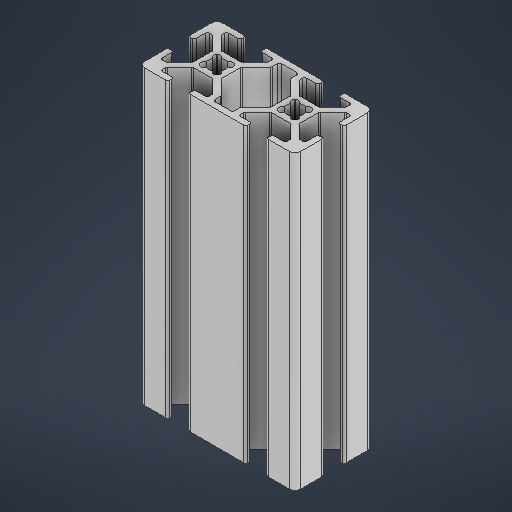
# Autodesk Inventor part: 20x40x100mm-Extrusion
Saved by Autodesk Inventor 2026.2 (Build 302298000, 298)
## iProperties
Created: 2026-06-17
Part Number: 20x40x100mm-Extrusion
Material: Aluminum 6061
Document SubType Name: Modeling
Designer: Kenji
Density: 2.7 g/cm^3
Appearance: Aluminum - Dark
Mass: 74.3604 g
Surface Area: 338.77 cm^2
Volume: 27.5409 cm^3
Author: Kenji
Autodesk Inventor part; units mm, degrees
ref_plane "YZ Plane" through (0, 0, 0) normal (1, 0, 0) x (0, 1, 0)
ref_plane "XZ Plane" through (0, 0, 0) normal (0, 1, 0) x (-1, 0, 0)
ref_plane "XY Plane" through (0, 0, 0) normal (0, 0, 1) x (1, 0, 0)
sketch "Sketch1" plane through (0, 0, 0) normal (0, 1, 0) x (-1, 0, 0)
  arc A0 (12.6651, -3.7453) -> (12.3059, -3.5965) centre (12.3059, -4.1045) ccw
  line L0 (15.7682, -6.8484) -> (12.6651, -3.7453)
  arc A1 (15.917, -7.2076) -> (15.7682, -6.8484) centre (15.409, -7.2076) ccw
  line L1 (15.917, -7.9335) -> (15.917, -7.2076)
  arc A2 (15.409, -8.4415) -> (15.917, -7.9335) centre (15.409, -7.9335) ccw
  line L2 (13.06, -8.4415) -> (15.409, -8.4415)
  arc A3 (13.06, -8.4415) -> (12.552, -8.9495) centre (13.06, -8.9495) ccw
  line L3 (12.552, -9.4335) -> (12.552, -8.9495)
  arc A4 (12.552, -9.4335) -> (13.06, -9.9415) centre (13.06, -9.4335) ccw
  line L4 (18.422, -9.9415) -> (13.06, -9.9415)
  arc A5 (18.422, -9.9415) -> (19.922, -8.4415) centre (18.422, -8.4415) ccw
  line L5 (19.922, -3.0795) -> (19.922, -8.4415)
  arc A6 (19.922, -3.0795) -> (19.414, -2.5715) centre (19.414, -3.0795) ccw
  line L6 (18.93, -2.5715) -> (19.414, -2.5715)
  arc A7 (18.93, -2.5715) -> (18.422, -3.0795) centre (18.93, -3.0795) ccw
  line L7 (18.422, -5.4285) -> (18.422, -3.0795)
  arc A8 (17.914, -5.9365) -> (18.422, -5.4285) centre (17.914, -5.4285) ccw
  line L8 (17.1881, -5.9365) -> (17.914, -5.9365)
  arc A9 (16.8289, -5.7877) -> (17.1881, -5.9365) centre (17.1881, -5.4285) ccw
  line L9 (13.7258, -2.6846) -> (16.8289, -5.7877)
  arc A10 (13.577, -2.3254) -> (13.7258, -2.6846) centre (14.085, -2.3254) ccw
  line L10 (13.577, 2.4424) -> (13.577, -2.3254)
  arc A11 (13.7258, 2.8016) -> (13.577, 2.4424) centre (14.085, 2.4424) ccw
  line L11 (16.8289, 5.9047) -> (13.7258, 2.8016)
  arc A12 (17.1881, 6.0535) -> (16.8289, 5.9047) centre (17.1881, 5.5455) ccw
  line L12 (17.914, 6.0535) -> (17.1881, 6.0535)
  arc A13 (18.422, 5.5455) -> (17.914, 6.0535) centre (17.914, 5.5455) ccw
  line L13 (18.422, 3.1965) -> (18.422, 5.5455)
  arc A14 (18.422, 3.1965) -> (18.93, 2.6885) centre (18.93, 3.1965) ccw
  line L14 (19.414, 2.6885) -> (18.93, 2.6885)
  arc A15 (19.414, 2.6885) -> (19.922, 3.1965) centre (19.414, 3.1965) ccw
  line L15 (19.922, 8.5585) -> (19.922, 3.1965)
  arc A16 (19.922, 8.5585) -> (18.422, 10.0585) centre (18.422, 8.5585) ccw
  line L16 (13.06, 10.0585) -> (18.422, 10.0585)
  arc A17 (13.06, 10.0585) -> (12.552, 9.5505) centre (13.06, 9.5505) ccw
  line L17 (12.552, 9.0665) -> (12.552, 9.5505)
  arc A18 (12.552, 9.0665) -> (13.06, 8.5585) centre (13.06, 9.0665) ccw
  line L18 (15.409, 8.5585) -> (13.06, 8.5585)
  arc A19 (15.917, 8.0505) -> (15.409, 8.5585) centre (15.409, 8.0505) ccw
  line L19 (15.917, 7.3246) -> (15.917, 8.0505)
  arc A20 (15.7682, 6.9654) -> (15.917, 7.3246) centre (15.409, 7.3246) ccw
  line L20 (12.6651, 3.8623) -> (15.7682, 6.9654)
  arc A21 (12.3059, 3.7135) -> (12.6651, 3.8623) centre (12.3059, 4.2215) ccw
  line L21 (7.5381, 3.7135) -> (12.3059, 3.7135)
  arc A22 (7.1789, 3.8623) -> (7.5381, 3.7135) centre (7.5381, 4.2215) ccw
  line L22 (4.0758, 6.9654) -> (7.1789, 3.8623)
  arc A23 (3.927, 7.3246) -> (4.0758, 6.9654) centre (4.435, 7.3246) ccw
  line L23 (3.927, 8.0505) -> (3.927, 7.3246)
  arc A24 (4.435, 8.5585) -> (3.927, 8.0505) centre (4.435, 8.0505) ccw
  line L24 (6.784, 8.5585) -> (4.435, 8.5585)
  arc A25 (6.784, 8.5585) -> (7.292, 9.0665) centre (6.784, 9.0665) ccw
  line L25 (7.292, 9.5505) -> (7.292, 9.0665)
  arc A26 (7.292, 9.5505) -> (6.784, 10.0585) centre (6.784, 9.5505) ccw
  line L26 (-6.94, 10.0585) -> (6.784, 10.0585)
  arc A27 (-6.94, 10.0585) -> (-7.448, 9.5505) centre (-6.94, 9.5505) ccw
  line L27 (-7.448, 9.0665) -> (-7.448, 9.5505)
  arc A28 (-7.448, 9.0665) -> (-6.94, 8.5585) centre (-6.94, 9.0665) ccw
  line L28 (-4.591, 8.5585) -> (-6.94, 8.5585)
  arc A29 (-4.083, 8.0505) -> (-4.591, 8.5585) centre (-4.591, 8.0505) ccw
  line L29 (-4.083, 7.3246) -> (-4.083, 8.0505)
  arc A30 (-4.2318, 6.9654) -> (-4.083, 7.3246) centre (-4.591, 7.3246) ccw
  line L30 (-7.3349, 3.8623) -> (-4.2318, 6.9654)
  arc A31 (-7.6941, 3.7135) -> (-7.3349, 3.8623) centre (-7.6941, 4.2215) ccw
  line L31 (-12.4619, 3.7135) -> (-7.6941, 3.7135)
  arc A32 (-12.8211, 3.8623) -> (-12.4619, 3.7135) centre (-12.4619, 4.2215) ccw
  line L32 (-15.9242, 6.9654) -> (-12.8211, 3.8623)
  arc A33 (-16.073, 7.3246) -> (-15.9242, 6.9654) centre (-15.565, 7.3246) ccw
  line L33 (-16.073, 8.0505) -> (-16.073, 7.3246)
  arc A34 (-15.565, 8.5585) -> (-16.073, 8.0505) centre (-15.565, 8.0505) ccw
  line L34 (-13.216, 8.5585) -> (-15.565, 8.5585)
  arc A35 (-13.216, 8.5585) -> (-12.708, 9.0665) centre (-13.216, 9.0665) ccw
  line L35 (-12.708, 9.5505) -> (-12.708, 9.0665)
  arc A36 (-12.708, 9.5505) -> (-13.216, 10.0585) centre (-13.216, 9.5505) ccw
  line L36 (-18.578, 10.0585) -> (-13.216, 10.0585)
  arc A37 (-18.578, 10.0585) -> (-20.078, 8.5585) centre (-18.578, 8.5585) ccw
  line L37 (-20.078, 3.1965) -> (-20.078, 8.5585)
  arc A38 (-20.078, 3.1965) -> (-19.57, 2.6885) centre (-19.57, 3.1965) ccw
  line L38 (-19.086, 2.6885) -> (-19.57, 2.6885)
  arc A39 (-19.086, 2.6885) -> (-18.578, 3.1965) centre (-19.086, 3.1965) ccw
  line L39 (-18.578, 5.5455) -> (-18.578, 3.1965)
  arc A40 (-18.07, 6.0535) -> (-18.578, 5.5455) centre (-18.07, 5.5455) ccw
  line L40 (-17.3441, 6.0535) -> (-18.07, 6.0535)
  arc A41 (-16.9849, 5.9047) -> (-17.3441, 6.0535) centre (-17.3441, 5.5455) ccw
  line L41 (-13.8818, 2.8016) -> (-16.9849, 5.9047)
  arc A42 (-13.733, 2.4424) -> (-13.8818, 2.8016) centre (-14.241, 2.4424) ccw
  line L42 (-13.733, -2.3254) -> (-13.733, 2.4424)
  arc A43 (-13.8818, -2.6846) -> (-13.733, -2.3254) centre (-14.241, -2.3254) ccw
  line L43 (-16.9849, -5.7877) -> (-13.8818, -2.6846)
  arc A44 (-17.3441, -5.9365) -> (-16.9849, -5.7877) centre (-17.3441, -5.4285) ccw
  line L44 (-18.07, -5.9365) -> (-17.3441, -5.9365)
  arc A45 (-18.578, -5.4285) -> (-18.07, -5.9365) centre (-18.07, -5.4285) ccw
  line L45 (-18.578, -3.0795) -> (-18.578, -5.4285)
  arc A46 (-18.578, -3.0795) -> (-19.086, -2.5715) centre (-19.086, -3.0795) ccw
  line L46 (-19.57, -2.5715) -> (-19.086, -2.5715)
  arc A47 (-19.57, -2.5715) -> (-20.078, -3.0795) centre (-19.57, -3.0795) ccw
  line L47 (-20.078, -8.4415) -> (-20.078, -3.0795)
  arc A48 (-20.078, -8.4415) -> (-18.578, -9.9415) centre (-18.578, -8.4415) ccw
  line L48 (-13.216, -9.9415) -> (-18.578, -9.9415)
  arc A49 (-13.216, -9.9415) -> (-12.708, -9.4335) centre (-13.216, -9.4335) ccw
  line L49 (-12.708, -8.9495) -> (-12.708, -9.4335)
  arc A50 (-12.708, -8.9495) -> (-13.216, -8.4415) centre (-13.216, -8.9495) ccw
  line L50 (-15.565, -8.4415) -> (-13.216, -8.4415)
  arc A51 (-16.073, -7.9335) -> (-15.565, -8.4415) centre (-15.565, -7.9335) ccw
  line L51 (-16.073, -7.2076) -> (-16.073, -7.9335)
  arc A52 (-15.9242, -6.8484) -> (-16.073, -7.2076) centre (-15.565, -7.2076) ccw
  line L52 (-12.8211, -3.7453) -> (-15.9242, -6.8484)
  arc A53 (-12.4619, -3.5965) -> (-12.8211, -3.7453) centre (-12.4619, -4.1045) ccw
  line L53 (-7.6941, -3.5965) -> (-12.4619, -3.5965)
  arc A54 (-7.3349, -3.7453) -> (-7.6941, -3.5965) centre (-7.6941, -4.1045) ccw
  line L54 (-4.2318, -6.8484) -> (-7.3349, -3.7453)
  arc A55 (-4.083, -7.2076) -> (-4.2318, -6.8484) centre (-4.591, -7.2076) ccw
  line L55 (-4.083, -7.9335) -> (-4.083, -7.2076)
  arc A56 (-4.591, -8.4415) -> (-4.083, -7.9335) centre (-4.591, -7.9335) ccw
  line L56 (-6.94, -8.4415) -> (-4.591, -8.4415)
  arc A57 (-6.94, -8.4415) -> (-7.448, -8.9495) centre (-6.94, -8.9495) ccw
  line L57 (-7.448, -9.4335) -> (-7.448, -8.9495)
  arc A58 (-7.448, -9.4335) -> (-6.94, -9.9415) centre (-6.94, -9.4335) ccw
  line L58 (6.784, -9.9415) -> (-6.94, -9.9415)
  arc A59 (6.784, -9.9415) -> (7.292, -9.4335) centre (6.784, -9.4335) ccw
  line L59 (7.292, -8.9495) -> (7.292, -9.4335)
  arc A60 (7.292, -8.9495) -> (6.784, -8.4415) centre (6.784, -8.9495) ccw
  line L60 (4.435, -8.4415) -> (6.784, -8.4415)
  arc A61 (3.927, -7.9335) -> (4.435, -8.4415) centre (4.435, -7.9335) ccw
  line L61 (3.927, -7.2076) -> (3.927, -7.9335)
  arc A62 (4.0758, -6.8484) -> (3.927, -7.2076) centre (4.435, -7.2076) ccw
  line L62 (7.1789, -3.7453) -> (4.0758, -6.8484)
  arc A63 (7.5381, -3.5965) -> (7.1789, -3.7453) centre (7.5381, -4.1045) ccw
  line L63 (12.3059, -3.5965) -> (7.5381, -3.5965)
  arc A64 (-9.274, -1.8766) -> (-7.9531, -2.246) centre (-8.5096, -1.6895) ccw
  arc A65 (-10.882, -1.8766) -> (-9.274, -1.8766) centre (-10.078, 0.0585) ccw
  arc A66 (-12.2029, -2.246) -> (-10.882, -1.8766) centre (-11.6464, -1.6895) ccw
  line L64 (-12.2029, -2.246) -> (-12.3825, -2.0664)
  arc A67 (-12.0131, -0.7455) -> (-12.3825, -2.0664) centre (-11.826, -1.5099) ccw
  arc A68 (-12.0131, 0.8625) -> (-12.0131, -0.7455) centre (-10.078, 0.0585) ccw
  arc A69 (-12.3825, 2.1834) -> (-12.0131, 0.8625) centre (-11.826, 1.6269) ccw
  line L65 (-12.3825, 2.1834) -> (-12.2029, 2.363)
  arc A70 (-10.882, 1.9936) -> (-12.2029, 2.363) centre (-11.6464, 1.8065) ccw
  arc A71 (-9.274, 1.9936) -> (-10.882, 1.9936) centre (-10.078, 0.0585) ccw
  arc A72 (-7.9531, 2.363) -> (-9.274, 1.9936) centre (-8.5096, 1.8065) ccw
  line L66 (-7.9531, 2.363) -> (-7.7735, 2.1834)
  arc A73 (-8.1429, 0.8625) -> (-7.7735, 2.1834) centre (-8.33, 1.6269) ccw
  arc A74 (-8.1429, -0.7455) -> (-8.1429, 0.8625) centre (-10.078, 0.0585) ccw
  arc A75 (-7.7735, -2.0664) -> (-8.1429, -0.7455) centre (-8.33, -1.5099) ccw
  line L67 (-7.7735, -2.0664) -> (-7.9531, -2.246)
  arc A76 (10.726, -1.8766) -> (12.0469, -2.246) centre (11.4904, -1.6895) ccw
  arc A77 (9.118, -1.8766) -> (10.726, -1.8766) centre (9.922, 0.0585) ccw
  arc A78 (7.7971, -2.246) -> (9.118, -1.8766) centre (8.3536, -1.6895) ccw
  line L68 (7.7971, -2.246) -> (7.6175, -2.0664)
  arc A79 (7.9869, -0.7455) -> (7.6175, -2.0664) centre (8.174, -1.5099) ccw
  arc A80 (7.9869, 0.8625) -> (7.9869, -0.7455) centre (9.922, 0.0585) ccw
  arc A81 (7.6175, 2.1834) -> (7.9869, 0.8625) centre (8.174, 1.6269) ccw
  line L69 (7.6175, 2.1834) -> (7.7971, 2.363)
  arc A82 (9.118, 1.9936) -> (7.7971, 2.363) centre (8.3536, 1.8065) ccw
  arc A83 (10.726, 1.9936) -> (9.118, 1.9936) centre (9.922, 0.0585) ccw
  arc A84 (12.0469, 2.363) -> (10.726, 1.9936) centre (11.4904, 1.8065) ccw
  line L70 (12.0469, 2.363) -> (12.2265, 2.1834)
  arc A85 (11.8571, 0.8625) -> (12.2265, 2.1834) centre (11.67, 1.6269) ccw
  arc A86 (11.8571, -0.7455) -> (11.8571, 0.8625) centre (9.922, 0.0585) ccw
  arc A87 (12.2265, -2.0664) -> (11.8571, -0.7455) centre (11.67, -1.5099) ccw
  line L71 (12.2265, -2.0664) -> (12.0469, -2.246)
  arc A88 (1.919, -8.4415) -> (2.427, -7.9335) centre (1.919, -7.9335) ccw
  line L72 (1.919, -8.4415) -> (-2.075, -8.4415)
  arc A89 (-2.583, -7.9335) -> (-2.075, -8.4415) centre (-2.075, -7.9335) ccw
  line L73 (-2.583, -7.9335) -> (-2.583, -6.5863)
  arc A90 (-2.583, -6.5863) -> (-2.7318, -6.227) centre (-3.091, -6.5863) ccw
  line L74 (-2.7318, -6.227) -> (-6.2742, -2.6846)
  arc A91 (-6.423, -2.3254) -> (-6.2742, -2.6846) centre (-5.915, -2.3254) ccw
  line L75 (-6.423, -2.3254) -> (-6.423, 2.4424)
  arc A92 (-6.2742, 2.8016) -> (-6.423, 2.4424) centre (-5.915, 2.4424) ccw
  line L76 (-6.2742, 2.8016) -> (-2.7318, 6.3441)
  arc A93 (-2.7318, 6.3441) -> (-2.583, 6.7033) centre (-3.091, 6.7033) ccw
  line L77 (-2.583, 6.7033) -> (-2.583, 8.0505)
  arc A94 (-2.075, 8.5585) -> (-2.583, 8.0505) centre (-2.075, 8.0505) ccw
  line L78 (-2.075, 8.5585) -> (1.919, 8.5585)
  arc A95 (2.427, 8.0505) -> (1.919, 8.5585) centre (1.919, 8.0505) ccw
  line L79 (2.427, 8.0505) -> (2.427, 6.7033)
  arc A96 (2.427, 6.7033) -> (2.5758, 6.3441) centre (2.935, 6.7033) ccw
  line L80 (2.5758, 6.3441) -> (6.1182, 2.8016)
  arc A97 (6.267, 2.4424) -> (6.1182, 2.8016) centre (5.759, 2.4424) ccw
  line L81 (6.267, 2.4424) -> (6.267, -2.3254)
  arc A98 (6.1182, -2.6846) -> (6.267, -2.3254) centre (5.759, -2.3254) ccw
  line L82 (6.1182, -2.6846) -> (2.5758, -6.227)
  arc A99 (2.5758, -6.227) -> (2.427, -6.5863) centre (2.935, -6.5863) ccw
  line L83 (2.427, -6.5863) -> (2.427, -7.9335)
  point P0 (0, 0)
  constraints: 200 point on circle, 168 end point, 100 centre point, 32 vertical, 28 horizontal, 409 other
extrude "Extrusion1" add sketch "Sketch1" along normal blind 75
sketch "Sketch2" plane through (-6.784, 0, 10.0585) normal (0, 0, 1) x (1, 0, 0)
  circle A0 centre (16.862, 10) radius 2.6
  line L0 (26.862, 0) -> (26.862, 75) projected
  line L1 (14.4781, 75) -> (19.2459, 75) projected
  circle A1 centre (-3.138, 10) radius 2.6
  line L2 (-13.138, 0) -> (-13.138, 75) projected
  line L3 (20, 0) -> (25.362, 0) projected
  point P0 (6.784, 0)
  dimension "d2" = 5.2
  dimension "d3" = 10
  dimension "d5" = 10
  dimension "d6" = 10
  constraints: 2 centre point, 1 equal radius, 1 horizontal alignment
  measures "d2" diameter of A0
  measures "d3" distance from line of A0.centre L0
  measures "d5" distance from line of L2 A1.centre
  measures "d6" distance from line of L3 A0.centre
extrude "Extrusion2" cut sketch "Sketch2" against normal through all
equation "\"d5\" = d3"
body "Solid1"
